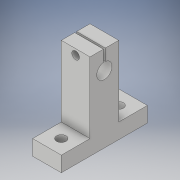
# Autodesk Inventor part: XRodClamp
Saved by Autodesk Inventor 2019 (Build 230136000, 136)
## iProperties
Created: 2019-08-18
Part Number: XRodClamp
Material: Generic
Document SubType Name: Modeling
Designer: Bruno
Density: 1 g/cm^3
Appearance: Default
Author: Bruno
Autodesk Inventor part; units mm, degrees
ref_plane "YZ Plane" through (0, 0, 0) normal (1, 0, 0) x (0, 1, 0)
ref_plane "XZ Plane" through (0, 0, 0) normal (0, 1, 0) x (-1, 0, 0)
ref_plane "XY Plane" through (0, 0, 0) normal (0, 0, 1) x (1, 0, 0)
sketch "Sketch1" plane through (0, 0, 0) normal (1, 0, 0) x (0, 1, 0)
  line L0 (-35, 22.5) -> (-35, -22.5)
  line L1 (-35, -22.5) -> (-27, -22.5)
  line L2 (-27, -22.5) -> (-27, -7.5)
  line L3 (-27, -7.5) -> (10, -7.5)
  line L4 (10, -7.5) -> (10, -0.5)
  line L5 (-35, 22.5) -> (-27, 22.5)
  line L6 (-27, 22.5) -> (-27, 7.5)
  line L7 (-27, 7.5) -> (10, 7.5)
  line L8 (10, 7.5) -> (10, 0.5)
  circle A0 centre (0, 0) radius 4
  line L9 (10, 0.5) -> (0, 0.5)
  line L10 (0, 0.5) -> (0, -0.5)
  line L11 (0, -0.5) -> (10, -0.5)
  line L12 (0, 0) -> (-20.797, 0) construction
  dimension "d0" = 8
  dimension "d1" = 1
  dimension "d2" = 7
  dimension "d3" = 15
  dimension "d5" = 37
  dimension "d6" = 8
  dimension "d11" = 35
  constraints: 26 end point, 9 perpendicular, 3 horizontal, 2 collinear, 1 centre point, 1 coincident, 1 midpoint, 1 vertical, 3 other
  measures "d0" diameter of A0
  measures "d1" distance between parallel lines of L11 L9
  measures "d2" distance of L3.end L4.end
  measures "d3" distance of L1.end L2.end
  measures "d5" distance of L6.end L7.end
  measures "d6" distance of L0.end L1.end
  measures "d11" distance from line of L0 L12.start
extrude "Extrusion1" add sketch "Sketch1" along normal blind 15 contours L5 L6 L7 L8 L9 A0 L11 L4 L3 L2 L1 L0 | L9 L10 L11 A0 picked at (-1.3236, -0.1605)
extrude "Extrusion2" cut sketch "Sketch1" along normal through all contours L9 L10 L11 A0 | A0 L11 L10 L9
sketch "Sketch2" plane through (0, -27, 22.5) normal (0, 1, 0) x (1, 0, 0)
  circle A0 centre (7.5, 7.5) radius 2.5
  circle A1 centre (7.5, 37.5) radius 2.5
  line L0 (0, 45) -> (0, 30) projected
  line L1 (0, 15) -> (0, 0) projected
  line L2 (0, 45) -> (0, 30) projected
  line L3 (0, 30) -> (15, 30) projected
  line L4 (15, 45) -> (15, 30) projected
  line L5 (0, 45) -> (15, 45) projected
  line L6 (0, 15) -> (0, 0) projected
  line L7 (0, 0) -> (15, 0) projected
  line L8 (15, 15) -> (15, 0) projected
  line L9 (0, 15) -> (15, 15) projected
  line L10 (7.5, 7.5) -> (0, 7.5)
  line L11 (0, 0) -> (0, 45) projected
  line L12 (7.5, 37.5) -> (15, 37.5)
  line L13 (15, 0) -> (15, 45) projected
  line L14 (7.5, 37.5) -> (0, 37.5)
  line L15 (7.5, 37.5) -> (7.5, 30)
  line L16 (7.5, 37.5) -> (7.5, 45)
  line L17 (0, 45) -> (15, 45) projected
  line L18 (7.5, 7.5) -> (15, 7.5)
  line L19 (7.5, 7.5) -> (7.5, 15)
  line L20 (0, 15) -> (15, 15) projected
  line L21 (7.5, 7.5) -> (7.5, 0)
  line L22 (0, 0) -> (15, 0) projected
  point P0 (0, 22.5)
  dimension "d12" = 5
  constraints: 16 end point, 5 midpoint, 5 point on line, 3 collinear, 2 centre point, 2 perpendicular, 2 vertical, 1 equal radius, 1 parallel, 2 other
  measures "d12" diameter of A0
extrude "Extrusion3" cut sketch "Sketch2" against normal through all contours L18 L19 A0 | A0 L21 L18 | L19 L10 A0 | A0 L10 L21 | L15 L12 A1 | A1 L14 L15 | L12 L16 A1 | A1 L16 L14
sketch "Sketch3" plane through (0, -27, 7.5) normal (0, 0, 1) x (1, 0, 0)
  circle A0 centre (7.5, 33.9843) radius 2
  line L0 (7.5, 33.9843) -> (0, 33.9843) construction
  line L1 (7.5, 33.9843) -> (15, 33.9843) construction
  line L2 (0, 37) -> (0, 0) projected
  line L3 (0, 37) -> (15, 37) projected
  line L4 (15, 30.9686) -> (15, 37) projected
  line L5 (15, 37) -> (15, 0) projected
  line L6 (7.5, 33.9843) -> (15, 37) construction
  line L7 (15, 30.9686) -> (15, 23) projected
  line L8 (15, 30.9686) -> (7.5, 33.9843) construction
  point P0 (0, 27)
  point P1 (15, 27)
  dimension "d15" = 4
  constraints: 8 end point, 2 equal length, 2 horizontal, 1 centre point, 1 point on line
  measures "d15" diameter of A0
extrude "Extrusion4" cut sketch "Sketch3" against normal through all
body "Solid1"
